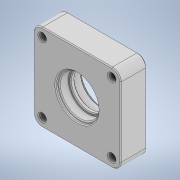
# Autodesk Inventor part: BearingBlockForPrototypePlate2
Saved by Autodesk Inventor 2020 (Build 240168000, 168)
## iProperties
Created: 2020-01-06
Part Number: BearingBlockForPrototypePlate2
Material: Generic
Document SubType Name: Modeling
Designer: srini
Density: 1 g/cm^3
Appearance: Default
Author: srini
Autodesk Inventor part; units mm, degrees
ref_plane "YZ Plane" through (0, 0, 0) normal (1, 0, 0) x (0, 1, 0)
ref_plane "XZ Plane" through (0, 0, 0) normal (0, 1, 0) x (-1, 0, 0)
sketch "Sketch1" plane through (0, 0, 0) normal (0, 0, 1) x (1, 0, 0)
  line L0 (-31.75, -31.75) -> (31.75, -31.75)
  line L1 (31.75, -31.75) -> (31.75, 31.75)
  line L2 (31.75, 31.75) -> (-31.75, 31.75)
  line L3 (-31.75, 31.75) -> (-31.75, -31.75)
  line L4 (-31.75, -31.75) -> (31.75, 31.75) construction
  line L5 (31.75, -31.75) -> (-31.75, 31.75) construction
  circle A0 centre (-25.4, 25.4) radius 2.5527
  circle A1 centre (25.4, 25.4) radius 2.5527
  circle A2 centre (-25.4, -25.4) radius 2.5527
  circle A3 centre (25.4, -25.4) radius 2.5527
  circle A4 centre (0, 0) radius 12.6746
  dimension "d0" = 63.5
  dimension "d1" = 63.5
  dimension "d2" = 6.35
  dimension "d5" = 50.8
  dimension "d8" = 50.8
  dimension "d11" = 5.1054
  dimension "d12" = 25.3492
  constraints: 12 end point, 5 centre point, 2 horizontal, 2 midpoint, 2 parallel, 1 coincident, 1 perpendicular, 1 point on line, 1 vertical, 6 other
  measures "d0" distance of L1.end L2.end
  measures "d1" distance of L2.end L0.start
  measures "d2" distance from line of A0.centre L3
  measures "d5" distance of A0.centre A1.centre
  measures "d8" distance of A0.centre A2.centre
  measures "d11" diameter of A0
  measures "d12" diameter of A4
extrude "Extrusion1" add sketch "Sketch1" along normal blind 19.05
fillet "Fillet1" radius 6.35 4 edges at (31.75, 31.75, 9.525) (31.75, -31.75, 9.525) (-31.75, -31.75, 9.525) (-31.75, 31.75, 9.525)
sketch "Sketch2" plane through (0, 0, 19.05) normal (0, 0, 1) x (1, 0, 0)
  circle A0 centre (0, 0) radius 14.3002
  dimension "d16" = 28.6004
  constraints: 1 centre point, 1 coincident
  measures "d16" diameter of A0
extrude "Extrusion2" cut sketch "Sketch2" against normal blind 7.9756
sketch "Sketch3" plane through (0, 0, 19.05) normal (0, 0, 1) x (1, 0, 0)
  circle A0 centre (0, 0) radius 15.5702
  dimension "d19" = 31.1404
  constraints: 1 centre point, 1 coincident
  measures "d19" diameter of A0
extrude "Extrusion3" cut sketch "Sketch3" against normal blind 1.6256
ref_plane "Work Plane1" through (0, 0, 9.525) normal (0, 0, 1) x (1, 0, 0)
mirror "Mirror1" about plane through (0, 0, 9.525) normal (0, 0, 1) of "Extrusion2", "Extrusion3"
chamfer "Chamfer1" distance 0.635 angle 45 16 edges at (-31.75, 0, 19.05) (-29.8901, -29.8901, 19.05) (0, -31.75, 19.05) (29.8901, -29.8901, 19.05) (31.75, 0, 19.05) (29.8901, 29.8901, 19.05) (0, 31.75, 19.05) (-29.8901, 29.8901, 19.05) (0, -31.75, 0) (29.8901, -29.8901, 0) (31.75, 0, 0) (29.8901, 29.8901, 0) (0, 31.75, 0) (-29.8901, 29.8901, 0) (-31.75, 0, 0) (-29.8901, -29.8901, 0)
chamfer "Chamfer2" distance 0.635 angle 45 6 edges at (-15.5702, 0, 19.05) (-14.3002, 0, 17.4244) (-12.6746, 0, 11.0744) (-12.6746, 0, 7.9756) (-14.3002, 0, 1.6256) (-15.5702, 0, 0)
chamfer "Chamfer3" distance 0.635 angle 45 8 edges at (-27.9527, -25.4, 19.05) (22.8473, -25.4, 19.05) (22.8473, 25.4, 19.05) (-27.9527, 25.4, 19.05) (22.8473, 25.4, 0) (22.8473, -25.4, 0) (-27.9527, -25.4, 0) (-27.9527, 25.4, 0)
body "Solid1"
